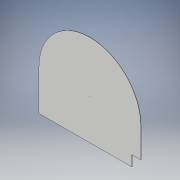
# Autodesk Inventor part: section
Saved by Autodesk Inventor 2019.4 (Build 234330000, 330)
## iProperties
Created: 2022-06-30
Part Number: section
Material: Generic
Document SubType Name: Modeling
Designer: mcgratta
Density: 1 g/cm^3
Appearance: Default
Author: mcgratta
Autodesk Inventor part; units mm, degrees
ref_plane "YZ Plane" through (0, 0, 0) normal (1, 0, 0) x (0, 1, 0)
ref_plane "XZ Plane" through (0, 0, 0) normal (0, 1, 0) x (-1, 0, 0)
ref_plane "XY Plane" through (0, 0, 0) normal (0, 0, 1) x (1, 0, 0)
sketch "Sketch1" plane through (0, 0, 0) normal (0, 0, 1) x (1, 0, 0)
  arc A0 (4389.12, 0) -> (-4389.12, 0) centre (0, 0) ccw
  line L0 (-4389.12, 0) -> (-4389.12, -3474.72)
  line L1 (-4389.12, -3474.72) -> (3627.12, -3474.72)
  line L2 (3627.12, -3474.72) -> (3627.12, -2560.32)
  line L3 (3627.12, -2560.32) -> (4389.12, -2560.32)
  line L4 (4389.12, -2560.32) -> (4389.12, 0)
  circle A1 centre (0, 0) radius 12.7
  dimension "d0" = 4389.12
  dimension "d1" = 3474.72
  dimension "d2" = 914.4
  dimension "d3" = 762
  dimension "d4" = 2560.32
  dimension "d5" = 8016.24
  dimension "d6" = 25.4
  constraints: 10 end point, 4 perpendicular, 2 centre point, 2 coincident, 2 point on circle, 1 vertical
  measures "d0" distance of point (0, 0) L0.start
  measures "d1" distance of L0.start L0.end
  measures "d2" distance of L1.end L2.end
  measures "d3" distance of L2.end L3.end
  measures "d4" distance of L3.end L4.end
  measures "d5" distance of L0.end L1.end
  measures "d6" diameter of A1
extrude "Extrusion1" add sketch "Sketch1" along normal blind 25.4
body "Solid1"
